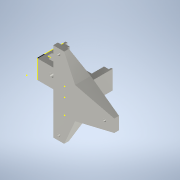
# Autodesk Inventor part: Part1
Saved by Autodesk Inventor 2022 (Build 260153000, 153)
## iProperties
Created: 2021-06-21
Part Number: Part1
Material: Silver
Document SubType Name: Modeling
Designer: Prajwal Patil
Density: 10.49 g/cm^3
Appearance: Silver
Author: Prajwal Patil
Autodesk Inventor part; units mm, degrees
sketch "Sketch1" plane through (0, 0, 0) normal (0, 0, 1) x (1, 0, 0)
  line L0 (-18.6207, 25.658) -> (16.9393, 25.658)
  line L1 (16.9393, 25.658) -> (16.9393, -25.142)
  line L2 (16.9393, -25.142) -> (-18.6207, -25.142)
  line L3 (-18.6207, -25.142) -> (-18.6207, 25.658)
  line L4 (-18.6207, 25.658) -> (24.5593, 25.658) construction
  line L5 (-18.6207, -25.142) -> (24.5593, -25.142) construction
  line L6 (-14.8574, -68.1577) -> (2.9226, -68.1577)
  line L7 (-14.8574, 68.6736) -> (2.9226, 68.6736)
  line L8 (16.9393, -25.142) -> (82.9793, -25.142) construction
  line L9 (16.9393, -25.142) -> (82.9793, -25.142) construction
  line L10 (16.9393, 25.658) -> (82.9793, 25.658) construction
  line L11 (81.7282, 12.8646) -> (81.7282, -12.3487)
  line L12 (16.9393, -25.142) -> (2.9226, -68.1577)
  line L13 (-18.6207, -25.142) -> (-14.8574, -68.1577)
  line L14 (-14.8574, 68.6736) -> (-18.6207, 25.658)
  line L15 (2.9226, 68.6736) -> (16.9393, 25.658)
  line L16 (81.7282, 12.8646) -> (16.9393, 25.658)
  line L17 (81.7282, -12.3487) -> (16.9393, -25.142)
  line L18 (-14.8574, 68.6736) -> (0.6798, 68.6736) construction
  point P0 (0, 0)
  dimension "d0" = 35.56
  dimension "d1" = 50.8
  dimension "d2" = 43.18
  dimension "d4" = 43.18
  dimension "d6" = 17.78
  dimension "d7" = 17.78
  dimension "d10" = 66.04
  dimension "d12" = 66.04
  constraints: 38 end point, 8 horizontal, 3 parallel, 1 perpendicular
  measures "d0" distance of L1.end L2.end
  measures "d1" distance of L0.end L1.end
  measures "d2" distance of L0.start L7.start
  measures "d4" distance of L2.end L6.start
  measures "d6" distance of L6.start L6.end
  measures "d7" distance of L7.start L7.end
  measures "d10" distance of L1.end L11.end
  measures "d12" distance of L0.end L11.start
extrude "Extrusion1" add sketch "Sketch1" against normal blind 25.4 contours L0 L1 L2 L3
ref_plane "Work Plane2" through (-18.6207, 63.758, 0) normal (0, 1, 0) x (1, 0, 0)
sketch "Sketch10" plane through (-18.6207, 63.758, 0) normal (0, 1, 0) x (1, 0, 0)
  line L0 (0, 0) -> (35.56, 0) projected
  line L1 (0, 0) -> (0, 7.62)
  line L2 (0, 0) -> (0, 25.4) projected
  line L3 (0, 7.62) -> (17.78, 7.62)
  line L4 (17.78, 7.62) -> (17.78, 0)
  line L5 (0, 0) -> (17.78, 0)
  point P0 (18.6207, 0)
  dimension "d28" = 7.62
  dimension "d29" = 17.78
  constraints: 8 end point, 1 collinear, 1 midpoint, 1 perpendicular, 1 point on line
  measures "d28" distance of L0.start L1.end
  measures "d29" distance of L1.end L3.end
loft "Loft1" add profiles "Sketch10" section 1 edges at (-0.8407, 25.658, 0) (16.9393, 25.658, -12.7) (-0.8407, 25.658, -25.4) (-18.6207, 25.658, -12.7)
ref_plane "Work Plane4" through (-18.6207, -65.782, 0) normal (0, -1, 0) x (1, 0, 0)
sketch "Sketch11" plane through (-18.6207, -25.142, 0) normal (0, -1, 0) x (1, 0, 0)
  point P0 (18.6207, 0)
sketch "Sketch12" plane through (-18.6207, -65.782, 0) normal (0, -1, 0) x (1, 0, 0)
  line L0 (0, 0) -> (35.56, 0) projected
  line L1 (17.78, -7.62) -> (0, -7.62) projected
  line L2 (0, 0) -> (17.78, 0)
  line L3 (17.78, 0) -> (17.78, -7.62)
  line L4 (17.78, -7.62) -> (0, -7.62)
  line L5 (0, -7.62) -> (0, 0)
  point P0 (18.6207, 0)
  constraints: 8 end point, 2 parallel, 1 horizontal, 1 perpendicular
loft "Loft2" add profiles "Sketch12" section 1 edges at (-0.8407, -25.142, 0) (-18.6207, -25.142, -12.7) (-0.8407, -25.142, -25.4) (16.9393, -25.142, -12.7)
ref_plane "Work Plane5" through (80.4393, 25.658, 0) normal (1, 0, 0) x (0, 0, -1)
sketch "Sketch13" plane through (80.4393, 25.658, 0) normal (1, 0, 0) x (0, 0, -1)
  line L0 (0, -15.2761) -> (7.62, -15.2761)
  line L1 (0, -35.5714) -> (7.62, -35.5714)
  line L2 (7.62, -35.5714) -> (7.62, -15.2761)
  line L3 (0, -15.2761) -> (0, -35.5714)
  point P0 (0, -25.658)
  dimension "d44" = 7.62
  constraints: 8 end point, 2 horizontal
  measures "d44" distance of L1.start L1.end
loft "Loft3" add profiles "Sketch13" section 1 edges at (16.9393, 0.258, 0) (16.9393, -25.142, -12.7) (16.9393, 0.258, -25.4) (16.9393, 25.658, -12.7)
sketch "Sketch17" plane through (0, 0, -25.4) normal (0, 0, -1) x (-1, 0, 0)
  line L0 (18.6207, 25.658) -> (-16.9393, 25.658) projected
  line L1 (-16.9393, 25.658) -> (-16.9393, -25.142) projected
  line L2 (-14.3993, 0.258) -> (-14.3993, -14.982)
  line L3 (-14.3993, -14.982) -> (18.6207, -14.982)
  line L4 (-14.3993, 0.258) -> (-14.3993, 15.498)
  line L5 (-14.3993, 15.498) -> (18.6207, 15.498)
  line L6 (-14.3993, -14.982) -> (61.8007, -14.982)
  line L7 (61.8007, -14.982) -> (61.8007, 15.498)
  line L8 (61.8007, 15.498) -> (-14.3993, 15.498)
  point P0 (0, 0)
  point P1 (18.6207, -25.142)
  dimension "d57" = 10.16
  dimension "d59" = 10.16
  dimension "d61" = 76.2
  constraints: 14 end point, 5 perpendicular, 1 point on line
  measures "d57" distance of point (18.621, -25.142) L3.end
  measures "d59" distance of L0.start L5.end
  measures "d61" distance of L2.end L6.end
extrude "Extrusion3" add sketch "Sketch17" along normal blind 38.1
sketch "Sketch18" plane through (0, 0, -63.5) normal (0, 0, -1) x (-1, 0, 0)
  line L0 (-14.3993, -14.982) -> (-14.3993, 15.498) projected
  line L1 (-14.3993, 15.498) -> (18.6207, 15.498) projected
  line L2 (-11.8593, 15.498) -> (-11.8593, -7.362)
  line L3 (-11.8593, -7.362) -> (-4.2393, -7.362)
  line L4 (61.8007, -14.982) -> (61.8007, 15.498) projected
  line L5 (59.2607, 15.498) -> (59.2607, -7.362)
  line L6 (59.2607, -7.362) -> (51.6407, -7.362)
  line L7 (51.6407, -7.362) -> (51.6407, -8.378)
  line L8 (-4.2393, -7.362) -> (-4.2393, -8.378)
  line L9 (-4.2393, -8.378) -> (51.6407, -8.378)
  line L10 (-14.3993, -14.982) -> (61.8007, -14.982) projected
  line L11 (59.2607, 15.498) -> (-11.8593, 15.498)
  point P0 (0, 0)
  point P1 (18.6207, 15.498)
  dimension "d64" = 2.54
  dimension "d66" = 7.62
  dimension "d67" = 2.54
  dimension "d68" = 7.62
  dimension "d69" = 1.016
  dimension "d70" = 1.016
  constraints: 16 end point, 3 vertical, 1 parallel, 1 perpendicular, 1 point on line
  measures "d64" distance of L0.end L2.start
  measures "d66" distance of L2.end L3.end
  measures "d67" distance of L4.end L5.start
  measures "d68" distance of L5.end L6.end
  measures "d69" distance of L6.end L7.end
  measures "d70" distance of L3.end L8.end
sketch "Sketch20" plane through (0, 0, -63.5) normal (0, 0, -1) x (-1, 0, 0)
  line L0 (61.8007, 15.498) -> (-14.3993, 15.498) projected
  line L1 (59.3978, 15.498) -> (-11.8609, 15.498)
  line L2 (-14.3993, 15.498) -> (18.6207, 15.498) projected
  point P0 (0, 0)
  constraints: 2 end point, 2 point on line
extrude "Extrusion4" cut sketch "Sketch18" against normal blind 38.1
sketch "Sketch21" plane through (0, 0, -25.4) normal (0, 0, 1) x (1, 0, 0)
  line L0 (-61.8007, 15.498) -> (-59.2607, 15.498) projected
  line L1 (-59.2607, 15.498) -> (-59.2607, -7.362)
  line L2 (-18.6207, -8.378) -> (-18.6207, 25.658) projected
  line L3 (-18.6207, 15.498) -> (-61.8007, 15.498)
  line L4 (-61.8007, -14.982) -> (-61.8007, 15.498) projected
  line L5 (-18.6207, -14.982) -> (-18.6207, -8.378) projected
  line L6 (-61.8007, -14.982) -> (-18.6207, -14.982)
  line L7 (-18.6207, -14.982) -> (-18.6207, 15.498)
  point P0 (0, 0)
  constraints: 8 end point, 2 perpendicular, 1 horizontal, 1 point on line, 1 vertical
extrude "Extrusion5" add sketch "Sketch21" along normal blind 8.382
sketch "Sketch22" plane through (0, 0, -25.4) normal (0, 0, -1) x (-1, 0, 0)
  line L0 (-11.8593, -7.362) -> (-11.8593, 15.498) projected
  line L1 (-4.2393, -7.362) -> (-11.8593, -7.362) projected
  line L2 (-11.8593, -7.362) -> (-4.2393, -7.362)
  line L3 (-4.2393, -7.362) -> (-4.2393, 15.498)
  line L4 (-4.2393, 15.498) -> (-11.8593, 15.498)
  point P0 (0, 0)
  dimension "d75" = 7.62
  constraints: 6 end point, 1 collinear, 1 perpendicular, 1 vertical
  measures "d75" distance of L0.start L1.start
extrude "Extrusion6" add sketch "Sketch22" along normal blind 34.29
sketch "Sketch23" plane through (0, 0, -25.4) normal (0, 0, -1) x (-1, 0, 0)
  line L0 (59.2607, -7.362) -> (51.6407, -7.362) projected
  line L1 (51.6407, -7.362) -> (59.2607, -7.362)
  line L2 (59.2607, -7.362) -> (59.2607, 15.498)
  line L3 (18.6207, 15.498) -> (61.8007, 15.498) projected
  line L4 (51.6407, -7.362) -> (51.6407, -8.378) projected
  line L5 (51.6407, 15.498) -> (51.6407, -7.362)
  line L6 (51.6407, -7.362) -> (59.2607, -7.362)
  point P0 (0, 0)
  constraints: 8 end point, 2 perpendicular, 1 collinear, 1 point on line, 1 vertical
extrude "Extrusion7" add sketch "Sketch23" along normal blind 34.29
sketch "Sketch24" plane through (-51.6407, 15.498, -25.4) normal (0, 1, 0) x (1, 0, 0)
  line L0 (0, 3.302) -> (-5.08, 3.302)
  line L1 (-5.08, 3.302) -> (-5.08, 10.922)
  line L2 (-5.08, 10.922) -> (0, 10.922)
  line L3 (0, 10.922) -> (0, 3.302)
  line L4 (0, 38.1) -> (0, 0) projected
  point P0 (51.6407, -25.4)
  dimension "d81" = 3.302
  dimension "d82" = 5.08
  dimension "d83" = 7.62
  constraints: 8 end point, 2 perpendicular, 1 collinear
  measures "d81" distance of L4.end L0.start
  measures "d82" distance of L0.start L0.end
  measures "d83" distance of L0.end L1.end
extrude "Extrusion8" cut sketch "Sketch24" against normal blind 16.51
sketch "Sketch26" plane through (-51.6407, 15.498, -25.4) normal (0, 1, 0) x (1, 0, 0)
  line L0 (0, 3.302) -> (-5.08, 3.302) projected
  point P0 (51.6407, -25.4)
sketch "Sketch27" plane through (-61.8007, -14.982, -63.5) normal (-1, 0, 0) x (0, 0, 1)
  point P0 (63.5, 14.982)
sketch "Sketch28" plane through (-61.8007, -14.982, -63.5) normal (-1, 0, 0) x (0, 0, 1)
  point P0 (63.5, 14.982)
sketch "Sketch29" plane through (-61.8007, -14.982, -63.5) normal (-1, 0, 0) x (0, 0, 1)
  line L0 (46.482, 30.48) -> (46.482, 0) projected
  line L1 (46.482, 30.48) -> (34.798, 30.48)
  line L2 (38.1, 30.48) -> (3.81, 30.48) projected
  point P0 (63.5, 14.982)
  constraints: 2 end point, 1 point on line
sketch "Sketch30" plane through (-61.8007, -14.982, -63.5) normal (-1, 0, 0) x (0, 0, 1)
  line L0 (38.1, 30.48) -> (3.81, 30.48) projected
  line L1 (46.482, 30.48) -> (34.7873, 30.48)
  line L2 (34.798, 24.892) -> (27.178, 24.892)
  line L3 (27.178, 24.892) -> (27.178, 13.462)
  line L4 (27.178, 13.462) -> (34.798, 13.462)
  line L5 (34.798, 24.892) -> (34.798, 13.462)
  point P0 (63.5, 14.982)
  dimension "d98" = 5.588
  dimension "d100" = 7.62
  dimension "d101" = 11.43
  constraints: 10 end point, 1 horizontal, 1 perpendicular, 1 point on line, 1 vertical
  measures "d98" distance of L1.end L2.start
  measures "d100" distance of L2.start L2.end
  measures "d101" distance of L2.end L3.end
extrude "Extrusion10" cut sketch "Sketch30" against normal blind 11.43
sketch "Sketch32" plane through (0, 0, 0) normal (0, 0, 1) x (1, 0, 0)
  line L0 (-18.6207, 63.758) -> (-18.6207, -65.782) projected
  line L1 (-18.6207, -65.782) -> (-0.8407, -65.782)
  line L2 (-0.8407, -65.782) -> (-9.7307, -65.782)
  circle A0 centre (-9.7307, -57.654) radius 2.54
  line L3 (-0.8407, 63.758) -> (-18.6207, 63.758) projected
  circle A1 centre (-9.7307, 55.63) radius 2.54
  line L4 (16.9393, -25.142) -> (80.4393, -9.9135) projected
  line L5 (80.4393, -9.9135) -> (80.4393, 10.3818) projected
  circle A2 centre (64.4373, 0.2342) radius 2.54
  point P0 (0, 0)
  dimension "d104" = 8.89
  dimension "d106" = 5.08
  dimension "d109" = 5.08
  dimension "d111" = 5.08
  constraints: 4 end point, 3 centre point, 1 horizontal, 1 midpoint
  measures "d104" distance of L1.end L2.end
  measures "d106" diameter of A0
  measures "d109" diameter of A1
  measures "d111" diameter of A2
extrude "Extrusion12" cut sketch "Sketch32" against normal through all
sketch "Sketch33" plane through (0, 0, -25.4) normal (0, 0, -1) x (-1, 0, 0)
  circle A0 centre (37.6707, 4.068) radius 3.81
  point P0 (0, 0)
  point P1 (51.6407, -7.362)
  dimension "d119" = 7.62
  constraints: 1 centre point
  measures "d119" diameter of A0
extrude "Extrusion13" cut sketch "Sketch33" against normal blind 25.4
sketch "Sketch34" plane through (0, 0, -59.69) normal (0, 0, -1) x (-1, 0, 0)
  line L0 (-4.2393, -7.362) -> (-11.8593, -7.362) projected
  line L1 (-11.8593, -7.362) -> (-11.8593, 4.068)
  line L2 (-11.8593, -7.362) -> (-11.8593, 15.498) projected
  line L3 (-11.8593, 4.068) -> (-8.0493, 4.068)
  line L4 (-8.0493, 4.068) -> (-8.0493, 10.164)
  line L5 (-8.0493, 4.068) -> (-8.0493, -2.028)
  circle A0 centre (-8.0493, -2.028) radius 1.27
  circle A1 centre (-8.0493, 10.164) radius 1.27
  line L6 (59.2607, 15.498) -> (59.2607, -7.362) projected
  line L7 (59.2607, -7.362) -> (59.2607, 4.068)
  line L8 (59.2607, 4.068) -> (55.4507, 4.068)
  line L9 (55.4507, 4.068) -> (55.4507, 10.164)
  line L10 (55.4507, 4.068) -> (55.4507, -2.028)
  circle A2 centre (55.4507, 10.164) radius 1.27
  circle A3 centre (55.4507, -2.028) radius 1.27
  point P0 (0, 0)
  dimension "d122" = 3.81
  dimension "d123" = 6.096
  dimension "d124" = 6.096
  dimension "d125" = 2.54
  dimension "d126" = 2.54
  dimension "d127" = 3.81
  dimension "d129" = 6.096
  dimension "d130" = 2.54
  dimension "d131" = 2.54
  constraints: 16 end point, 4 centre point, 4 coincident, 3 perpendicular, 3 vertical, 1 midpoint
  measures "d122" distance of L1.end L3.end
  measures "d123" distance of L3.end L4.end
  measures "d124" distance of L3.end L5.end
  measures "d125" diameter of A0
  measures "d126" diameter of A1
  measures "d127" distance of L7.end L8.end
  measures "d129" distance of L8.end L10.end
  measures "d130" diameter of A2
  measures "d131" diameter of A3
extrude "Extrusion14" cut sketch "Sketch34" against normal blind 10.16
sketch "Sketch35" plane through (0, 0, 0) normal (0, 0, 1) x (1, 0, 0)
  point P0 (0, 0)
body "Solid1"
